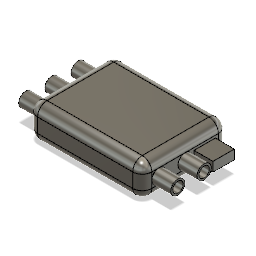
Electric connector v0 (Autodesk Fusion 360 design; units mm, degrees)
Autodesk Fusion 360 part; units mm, degrees
sketch "Sketch1" plane through (0, 0, 0) normal (0, 1, 0) x (1, 0, 0)
  line L0 (12, -9) -> (-12, -9)
  line L1 (-12, -9) -> (-12, 9)
  line L2 (-12, 9) -> (12, 9)
  line L3 (12, 9) -> (12, -9)
  line L4 (12, -9) -> (-12, 9) construction
  line L5 (-12, -9) -> (12, 9) construction
  dimension "d1" = 24
  dimension "d2" = 18
  constraint horizontal L0
  constraint perpendicular L0 L1
  constraint parallel L0 L2
  constraint parallel L1 L3
  constraint coincident L4 origin
  constraint coincident L5 origin
  measures "d1" distance of L1.end L2.end
  measures "d2" distance of L0.end L1.end
extrude "Extrude1" add sketch "Sketch1" along normal blind 7
fillet "Fillet1" radius 2 12 edges at (-12, 3.5, 9) (0, 7, 9) (0, 0, 9) (12, 3.5, 9) (12, 7, 0) (12, 0, 0) (12, 3.5, -9) (0, 7, -9) (0, 0, -9) (-12, 3.5, -9) (-12, 7, 0) (-12, 0, 0)
sketch "Sketch2" plane through (-12, 0, 0) normal (-1, 0, 0) x (0, 0, 1)
  line L0 (-7, 2) -> (7, 2)
  line L1 (7, 2) -> (7, 5)
  line L2 (7, 5) -> (-7, 5)
  line L3 (-7, 5) -> (-7, 2)
  line L4 (-7, 3.5) -> (7, 3.5) construction
  circle A0 centre (0, 3.5) radius 1.5
  circle A1 centre (0, 3.5) radius 1.1
  circle A2 centre (-5.5, 3.5) radius 1.5
  circle A3 centre (5.5, 3.5) radius 1.5
  circle A4 centre (5.5, 3.5) radius 1.1
  circle A5 centre (-5.5, 3.5) radius 1.1
  dimension "d6" = 2.2
  constraint midpoint L3 L4.start
  constraint midpoint L1 L4.end
  constraint midpoint L4 A0.centre
  constraint tangent L0 A0
  constraint concentric A0 A1
  constraint coincident L4 A2.centre
  constraint coincident L4.start A2
  constraint coincident L4 A3.centre
  constraint coincident L4.end A3
  constraint concentric A3 A4
  constraint equal A0 A2
  constraint equal A2 A3
  constraint equal A1 A4
  constraint concentric A2 A5
  constraint equal A1 A5
  measures "d6" diameter of A1
extrude "Extrude2" add sketch "Sketch2" along normal blind 4 contours A2 | A0 | A3
sketch "Sketch3" plane through (12, 0, 0) normal (1, 0, 0) x (0, 0, -1)
  line L0 (-7, 2) -> (7, 2)
  line L1 (7, 2) -> (7, 5)
  line L2 (7, 5) -> (-7, 5)
  line L3 (-7, 5) -> (-7, 2)
  line L4 (7, 3.5) -> (-7, 3.5) construction
  line L5 (6.3632, 4.5) -> (1.8632, 4.5)
  line L6 (1.8632, 4.5) -> (1.8632, 2.5)
  line L7 (1.8632, 2.5) -> (6.3632, 2.5)
  line L8 (6.3632, 2.5) -> (6.3632, 4.5)
  line L9 (6.3632, 4.5) -> (1.8632, 2.5) construction
  line L10 (1.8632, 4.5) -> (6.3632, 2.5) construction
  circle A0 centre (-5.5, 3.5) radius 1.5
  circle A1 centre (-5.5, 3.5) radius 1.1
  circle A2 centre (0, 3.5) radius 1.5
  circle A3 centre (0, 3.5) radius 1.1
  point P0 (4.1132, 3.5)
  dimension "d10" = 4.5
  dimension "d11" = 1
  dimension "d12" = 3
  dimension "d13" = 2.2
  constraint midpoint L1 L4.start
  constraint midpoint L3 L4.end
  constraint horizontal L5
  constraint perpendicular L5 L6
  constraint parallel L5 L7
  constraint parallel L6 L8
  constraint coincident L9 P0
  constraint coincident L10 P0
  constraint coincident L4 P0
  constraint coincident L4 A0.centre
  constraint coincident L4.end A0
  constraint concentric A0 A1
  constraint midpoint L4 A2.centre
  constraint concentric A2 A3
  constraint equal A0 A2
  constraint equal A1 A3
  measures "d10" distance of L6.end L7.end
  measures "d11" distance of L4 L5.start
  measures "d12" diameter of A0
  measures "d13" diameter of A1
extrude "Extrude3" add sketch "Sketch3" along normal blind 4 contours A0 | A2 | L5 L6 L7 L8
